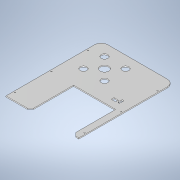
# Autodesk Inventor part: obudowa_zewnetrzna_tyl_korba
Saved by Autodesk Inventor 2020 (Build 240168000, 168)
## iProperties
Created: 2020-08-30
Part Number: obudowa_zewnetrzna_tyl_korba
Material: ABS Plastic
Document SubType Name: Sheet Metal
Designer: Hesekiel
Density: 1.06 g/cm^3
Appearance: Smooth - White
Sheet Metal Rule: Default
Author: Hesekiel
Autodesk Inventor part; units mm, degrees
ref_plane "YZ Plane" through (0, 0, 0) normal (1, 0, 0) x (0, 1, 0)
ref_plane "XZ Plane" through (0, 0, 0) normal (0, 1, 0) x (-1, 0, 0)
ref_plane "XY Plane" through (0, 0, 0) normal (0, 0, 1) x (1, 0, 0)
sketch "Sketch1" plane through (0, 0, 0) normal (0, 1, 0) x (-1, 0, 0)
  line L0 (-132.5, 287.3805) -> (-122.5, 287.3805)
  line L1 (-132.5, 20) -> (-132.5, 287.3805)
  line L2 (-122.5, 20) -> (-122.5, 287.3805)
  line L3 (77.5, 287.3805) -> (87.5, 287.3805)
  line L4 (77.5, 20) -> (77.5, 287.3805)
  line L5 (87.5, 20) -> (87.5, 287.3805)
  line L6 (82.5, 0) -> (127.5, 0) construction
  line L7 (-132.5, 20) -> (-132.5, 287.3805)
  line L8 (82.5, 45) -> (-127.5, 45)
  line L9 (82.5, 155) -> (-127.5, 155)
  circle A0 centre (-127.5, 265) radius 1.6
  circle A1 centre (-127.5, 155) radius 1.6
  circle A2 centre (-127.5, 45) radius 1.6
  circle A3 centre (82.5, 45) radius 1.6
  circle A4 centre (82.5, 155) radius 1.6
  circle A5 centre (82.5, 265) radius 1.6
  line L10 (-132.5, 287.3805) -> (87.5, 287.3805)
  line L11 (87.5, 287.3805) -> (87.5, 0)
  line L12 (87.5, 0) -> (-132.5, 0)
  line L13 (-132.5, 0) -> (-132.5, 287.3805)
  line L14 (87.5, 0) -> (-132.5, 0)
  line L15 (-132.5, 0) -> (-132.5, -22.8)
  line L16 (-132.5, -22.8) -> (87.5, -22.8)
  line L17 (87.5, -22.8) -> (87.5, 0)
  arc A6 (6, 100) -> (0, 94) centre (6, 94) ccw
  line L18 (0, 0) -> (0, 94)
  line L19 (0, 0) -> (90, 0)
  line L20 (90, 0) -> (90, 94)
  arc A7 (90, 94) -> (84, 100) centre (84, 94) ccw
  line L21 (6, 100) -> (84, 100)
  circle A8 centre (45, 47.3805) radius 11
  circle A9 centre (76.75, 79.1305) radius 5.75
  circle A10 centre (13.25, 15.6305) radius 5.75
  circle A11 centre (76.75, 15.6305) radius 5.75
  circle A12 centre (13.25, 79.1305) radius 5.75
  circle A13 centre (117.5, 135) radius 1.8
  line L22 (112.5, 267.3805) -> (122.5, 267.3805)
  line L23 (112.5, 0) -> (112.5, 267.3805)
  line L24 (112.5, 0) -> (122.5, 0)
  line L25 (122.5, 0) -> (122.5, 267.3805)
  circle A14 centre (117.5, 25) radius 1.8
  circle A15 centre (117.5, 245) radius 1.8
  circle A16 centre (-92.5, 135) radius 1.8
  line L26 (-97.5, 267.3805) -> (-87.5, 267.3805)
  line L27 (-97.5, 0) -> (-97.5, 267.3805)
  line L28 (-97.5, 0) -> (-87.5, 0)
  line L29 (-87.5, 0) -> (-87.5, 267.3805)
  circle A17 centre (-92.5, 245) radius 1.8
  circle A18 centre (-92.5, 25) radius 1.8
  point P0 (-62.5, 0)
  point P1 (52.5, -20)
  dimension "d0" = 45
  dimension "d2" = 110
  dimension "d4" = 3.2
  dimension "d5" = 3.2
  dimension "d6" = 3.2
  dimension "d7" = 3.2
  dimension "d8" = 3.2
  dimension "d9" = 3.2
  dimension "d12" = 22.8
  constraints: 60 end point, 19 centre point, 4 coincident, 4 parallel, 4 point on circle, 3 horizontal, 2 perpendicular, 1 point on line
  measures "d0" distance of L6.start L8.start
  measures "d2" distance of L8.start L9.start
  measures "d4" diameter of A0
  measures "d5" diameter of A1
  measures "d6" diameter of A2
  measures "d7" diameter of A3
  measures "d8" diameter of A4
  measures "d9" diameter of A5
  measures "d12" distance of L15.end L14.end
extrude "Extrusion1" add sketch "Sketch1" along normal blind 3 contours L0 L2 L8 L27 L12 L13 L1 | L10 L4 L9 L29 L26 L27 L2 | L9 L27 L8 L2 | L3 L5 A7 L21 L4 | L27 L26 L29 L9 | L9 L29 L8 L27 | L4 L21 A6 L18 L8 L29 L9 | L27 L8 L29 L12 | L5 L11 L12 L18 L8 A8 L4 A9 L21 A7 | L4 A9 L8 A8 L18 A6 L21 | L29 L8 L18 L12 | A9 L4 | L4 A9 | A8 L8 | L8 A8 | A10 | A11 | A12 | A16 | A17 | A18
fillet "Fillet1" radius 20 2 edges at (132.5, 1.5, 0) (-87.5, 1.5, 0)
sketch "Sketch4" plane through (0, 0, 0) normal (0, -1, 0) x (1, 0, 0)
  line L0 (68.5, 205.2102) -> (31.5, 205.2102)
  line L1 (78.5, 192.2868) -> (21.5, 192.2868)
  line L2 (21.5, 205.2102) -> (31.5, 205.2102)
  line L3 (68.5, 205.2102) -> (78.5, 205.2102)
  line L4 (78.5, 205.2102) -> (78.5, 192.2868)
  line L5 (21.5, 192.2868) -> (21.5, 205.2102)
  circle A0 centre (21.75, 99.1305) radius 7.65
  circle A1 centre (-41.75, 99.1305) radius 7.65
  circle A2 centre (21.75, 35.6305) radius 7.65
  arc A3 (10, 67.3805) -> (-30, 67.3805) centre (-10, 67.3805) ccw
  line L6 (10, 67.3805) -> (10, -32.6195)
  line L7 (-30, -32.6195) -> (-30, 67.3805)
  circle A4 centre (-41.75, 35.6305) radius 7.65
  line L8 (-87.5, 20) -> (-87.5, 287.3805)
  line L9 (-87.5, 287.3805) -> (132.5, 287.3805)
  line L10 (132.5, 287.3805) -> (132.5, 20)
  line L11 (112.5, 0) -> (-67.5, 0)
  line L12 (-87.5, 20) -> (-87.5, 287.3805) projected
  line L13 (-87.5, 287.3805) -> (132.5, 287.3805) projected
  circle A5 centre (-41.75, 99.1305) radius 10
  circle A6 centre (21.75, 99.1305) radius 10
  circle A7 centre (-41.75, 35.6305) radius 10
  circle A8 centre (21.75, 35.6305) radius 10
  line L14 (-87.5, 287.3805) -> (132.5, 287.3805) projected
  line L15 (21.75, 287.3805) -> (78.5, 287.3805)
  line L16 (78.5, 287.3805) -> (78.5, 157.3805)
  line L17 (78.5, 157.3805) -> (21.75, 157.3805)
  line L18 (21.75, 157.3805) -> (21.75, 287.3805)
  circle A9 centre (-10, 67.3805) radius 13
  line L19 (80.125, 157.3805) -> (20.125, 157.3805)
  line L20 (20.125, 157.3805) -> (20.125, 287.3805)
  line L21 (20.125, 287.3805) -> (80.125, 287.3805)
  line L22 (80.125, 287.3805) -> (80.125, 157.3805)
  line L23 (80.125, 157.3805) -> (20.125, 287.3805) construction
  line L24 (20.125, 157.3805) -> (80.125, 287.3805) construction
  line L25 (-13.375, 287.3805) -> (113.625, 287.3805)
  line L26 (113.625, 287.3805) -> (113.625, 157.3805)
  line L27 (113.625, 157.3805) -> (-13.375, 157.3805)
  line L28 (-13.375, 157.3805) -> (-13.375, 287.3805)
  line L29 (-13.375, 287.3805) -> (113.625, 157.3805) construction
  line L30 (113.625, 287.3805) -> (-13.375, 157.3805) construction
  point P0 (0, 0)
  point P1 (50.125, 222.3805)
  dimension "d24" = 20
  dimension "d25" = 20
  dimension "d26" = 20
  dimension "d27" = 20
  dimension "d28" = 130
  dimension "d29" = 26
  dimension "d36" = 60
  dimension "d37" = 130
  dimension "d38" = 127
  constraints: 56 end point, 10 centre point, 6 parallel, 5 coincident, 4 midpoint, 3 horizontal, 3 perpendicular, 2 point on circle, 1 point on line
  measures "d24" diameter of A5
  measures "d25" diameter of A6
  measures "d26" diameter of A7
  measures "d27" diameter of A8
  measures "d28" distance of L15.end L16.end
  measures "d29" diameter of A9
  measures "d36" distance of L20.end L21.end
  measures "d37" distance of L19.end L20.end
  measures "d38" distance of L26.end L27.end
extrude "Extrusion3" cut sketch "Sketch4" against normal up to surface (3 mm away) contours L3 L4 L1 L18 L2 L0 | L0 L2 L18 L9 L16 L3 | L16 L9 L22 L19 L4 | L18 L1 L5 L2 | L2 L5 L1 L18 L19 L20 L9 | L16 L17 L18 L1 | L9 L26 L27 L22 | L20 L27 L28 L9 | A0 | A1 | A2 | A4 | A5 | A6 | A7 | A8 | A9
chamfer "Chamfer1" distance 10 angle 45 2 edges at (-13.375, 1.5, 287.3805) (113.625, 1.5, 287.3805)
sketch "Sketch5" plane through (0, 0, 0) normal (0, -1, 0) x (1, 0, 0)
  line L0 (113.625, 157.3805) -> (-13.375, 157.3805) projected
  line L1 (113.625, 157.3805) -> (93.625, 157.3805)
  line L2 (93.625, 157.3805) -> (93.625, 137.3805)
  line L3 (93.625, 137.3805) -> (80.325, 137.3805)
  line L4 (80.325, 137.3805) -> (80.325, 128.8805)
  line L5 (80.325, 128.8805) -> (93.625, 128.8805)
  line L6 (93.625, 128.8805) -> (93.625, 137.3805)
  line L7 (93.625, 133.1305) -> (100.625, 133.1305)
  circle A0 centre (100.625, 133.1305) radius 3
  line L8 (97.625, 133.1305) -> (97.625, 127.1305)
  line L9 (103.625, 133.1305) -> (103.625, 127.1305)
  line L10 (100.625, 133.1305) -> (100.625, 124.1305)
  circle A1 centre (100.625, 124.1305) radius 3
  line L11 (97.625, 127.1305) -> (97.625, 124.1305)
  line L12 (103.625, 127.1305) -> (103.625, 124.1305)
  point P0 (0, 0)
  dimension "d39" = 20
  dimension "d40" = 20
  dimension "d41" = 13.3
  dimension "d42" = 8.5
  dimension "d45" = 7
  dimension "d46" = 6
  dimension "d47" = 6
  dimension "d48" = 6
  dimension "d49" = 9
  constraints: 24 end point, 4 point on circle, 4 tangent, 3 perpendicular, 2 centre point, 2 coincident, 2 horizontal, 2 parallel, 2 point on line, 2 vertical, 1 midpoint
  measures "d39" distance of L0.start L1.end
  measures "d40" distance of L1.end L2.end
  measures "d41" distance of L5.end L4.end
  measures "d42" distance of L4.end L3.end
  measures "d45" distance of L7.start L7.end
  measures "d46" diameter of A0
  measures "d47" distance of L8.start L8.end
  measures "d48" distance of L9.start L9.end
  measures "d49" distance of L10.start L10.end
extrude "Extrusion4" cut sketch "Sketch5" against normal up to surface (3 mm away)
equation "\"BendRadius\" = Thickness"
equation "\"BendReliefWidth\" = Thickness"
equation "\"BendReliefDepth\" = 0.5 * Thickness"
equation "\"CornerReliefSize\" = 4 * Thickness"
equation "\"MinimumRemnant\" = 2 * Thickness"
equation "\"TransitionRadius\" = BendRadius"
equation "\"JacobiRadiusSize\" = Thickness"
equation "\"GapSize\" = Thickness"
equation "\"Thickness\" = 0.5"
body "Solid1"
